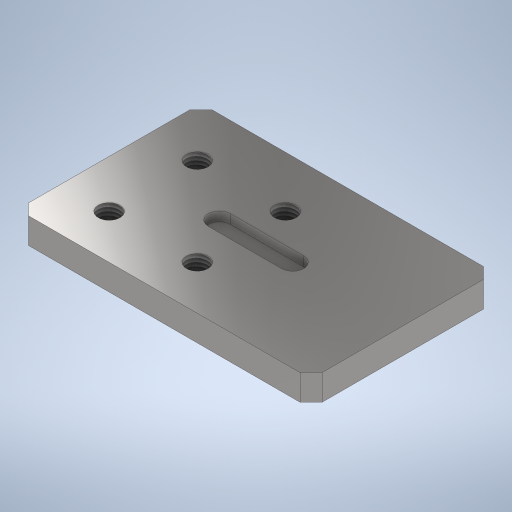
# Autodesk Inventor part: variante-03
Saved by Autodesk Inventor 2024 (Build 280153000, 153)
## iProperties
Created: 2024-02-21
Part Number: variante-03
Material: Edelstahl
Document SubType Name: Modeling
Designer: ffogue
Density: 8 g/cm^3
Appearance: Halbpoliert
Author: ffogue
Autodesk Inventor part; units mm, degrees
ref_plane "YZ Plane" through (0, 0, 0) normal (1, 0, 0) x (0, 1, 0)
ref_plane "XZ Plane" through (0, 0, 0) normal (0, 1, 0) x (-1, 0, 0)
ref_plane "XY Plane" through (0, 0, 0) normal (0, 0, 1) x (1, 0, 0)
sketch "Skizze1" plane through (0, 0, 0) normal (0, 0, 1) x (1, 0, 0)
  line L0 (0, 0) -> (80, 0)
  line L1 (80, 0) -> (80, 50)
  line L2 (80, 50) -> (0, 50)
  line L3 (0, 50) -> (0, 0)
  dimension "Breite" = 50
  dimension "Laenge" = 80
  constraints: 8 end point, 2 parallel, 1 horizontal, 1 perpendicular
  measures "Breite" distance between parallel lines of L0 L2
  measures "Laenge" distance between parallel lines of L1 L3
extrude "Extrusion1" add sketch "Skizze1" along normal blind 7
chamfer "Fasen1" distance 3 angle 45 4 edges at (80, 50, 3.5) (80, 0, 3.5) (0, 50, 3.5) (0, 0, 3.5)
sketch "Skizze2" plane through (0, 0, 7) normal (0, 0, 1) x (1, 0, 0)
  line L0 (77, 50) -> (3, 50) projected
  line L1 (40, 50) -> (40, 0) construction
  line L2 (0, 47) -> (0, 3) projected
  line L3 (0, 25) -> (80, 25) construction
  line L4 (80, 3) -> (80, 47) projected
  point P0 (0, 0)
  point P1 (13, 36)
  dimension "Punktabstand1" = 13
  dimension "Punktabstand2" = 14
  constraints: 4 end point, 3 midpoint, 1 vertical
  measures "Punktabstand1" distance from line of point (13, 36) L2
  measures "Punktabstand2" distance from line of point (13, 36) L0
hole "Bohrung1" at (13, 36, 7) direction (0, 0, -1) diameter 5.9175 end through all thread size "M7x1" class "6H" standard "ISO Metric profile"
sketch "Skizze3" plane through (0, 0, 7) normal (0, 0, 1) x (1, 0, 0)
  line L0 (30, 25) -> (50, 25) construction
  line L1 (30, 22) -> (50, 22)
  line L2 (50, 28) -> (30, 28)
  arc A0 (30, 28) -> (30, 22) centre (30, 25) ccw
  arc A1 (50, 22) -> (50, 28) centre (50, 25) ccw
  line L3 (3, 0) -> (77, 0) projected
  line L4 (0, 47) -> (0, 3) projected
  point P0 (0, 0)
  point P1 (40, 25)
  point P2 (40, 0)
  point P3 (0, 25)
  point P4 (40, 0)
  point P5 (0, 25)
  dimension "Mannlochbreite" = 6
  dimension "Mannlochlaenge" = 20
  constraints: 8 end point, 5 midpoint, 4 point on circle, 4 tangent, 2 centre point, 2 horizontal alignment, 2 vertical alignment, 1 horizontal, 1 parallel
  measures "Mannlochbreite" distance between parallel lines of L1 L2
  measures "Mannlochlaenge" distance of L1.start L1.end
extrude "Extrusion2" cut sketch "Skizze3" against normal blind 2.5
pattern_linear "Rechteckige Anordnung2" count 2 spacing 24 along (0, -1, 0) count 2 spacing 24 along (1, 0, 0) of "Bohrung1"
equation "\"d27\" = Abstand_Zeilen"
equation "\"d30\" = Abstand_Zeilen"
equation "\"Abstand_Zeilen\" = Breite - 2 * Punktabstand1"
equation "\"Abstand_Spalten\" = Laenge - 2 * Punktabstand2"
